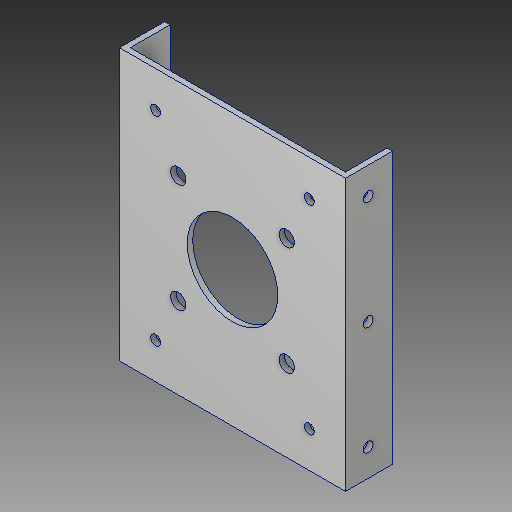
# Autodesk Inventor part: Pneumatic Connector
Saved by Autodesk Inventor 2019 (Build 230136000, 136)
## iProperties
Created: 2019-10-25
Part Number: Pneumatic Connector
Material: Aluminum 6061
Document SubType Name: Modeling
Designer: Mark
Density: 2.7 g/cm^3
Appearance: Aluminum - Flat
Mass: 129.385 g
Surface Area: 498.83 cm^2
Volume: 47.9204 cm^3
Author: Mark
Autodesk Inventor part; units mm, degrees
ref_plane "YZ Plane" through (0, 0, 0) normal (1, 0, 0) x (0, 1, 0)
ref_plane "XZ Plane" through (0, 0, 0) normal (0, 1, 0) x (-1, 0, 0)
ref_plane "XY Plane" through (0, 0, 0) normal (0, 0, 1) x (1, 0, 0)
sketch "Sketch1" plane through (0, 0, 0) normal (0, 1, 0) x (-1, 0, 0)
  line L0 (0, 0) -> (125, 0)
  line L1 (0, 0) -> (125, 0) construction
  line L2 (125, 0) -> (125, -25)
  line L3 (125, -25) -> (122, -25)
  line L4 (122, -25) -> (122, -3)
  line L5 (122, -3) -> (3, -3)
  line L6 (3, -3) -> (3, -26)
  line L7 (3, -26) -> (0, -26)
  line L8 (0, -26) -> (0, 0)
  dimension "d0" = 125
  dimension "d2" = 25
  dimension "d3" = 90
  dimension "d4" = 90
  dimension "d5" = 3
  dimension "d6" = 22
  dimension "d7" = 119
  dimension "d8" = 90
  dimension "d9" = 23
  dimension "d10" = 90
  dimension "d11" = 3
  dimension "d12" = 90
  constraints: 18 end point, 4 perpendicular, 2 horizontal, 1 collinear, 1 vertical
  measures "d0" distance of L0.start L0.end
  measures "d2" distance of L0.end L2.end
  measures "d3" angle of L0 L2
  measures "d4" angle of L3 L2
  measures "d5" distance of L2.end L3.end
  measures "d6" distance of L3.end L4.end
  measures "d7" distance of L4.end L5.end
  measures "d8" angle of L5 L4
  measures "d9" distance of L5.end L6.end
  measures "d10" angle of L6 L5
  measures "d11" distance of L6.end L7.end
  measures "d12" angle of L6 L7
extrude "Extrusion1" add sketch "Sketch1" along normal blind 150
sketch "Sketch2" plane through (-125, 0, 0) normal (0, 0, 1) x (1, 0, 0)
  circle A0 centre (32.5, 105) radius 4.25
  circle A1 centre (92.5, 105) radius 4.25
  circle A2 centre (32.5, 45) radius 4.25
  circle A3 centre (92.5, 45) radius 4.25
  line L0 (125, 0) -> (125, 150) projected
  line L1 (125, 0) -> (0, 0) projected
  circle A4 centre (62.5, 75) radius 25
  dimension "d15" = 8.5
  dimension "d16" = 8.5
  dimension "d17" = 8.5
  dimension "d18" = 8.5
  dimension "d19" = 60
  dimension "d20" = 60
  dimension "d21" = 60
  dimension "d22" = 60
  dimension "d23" = 60
  dimension "d24" = 60
  dimension "d25" = 32.5
  dimension "d26" = 45
  dimension "d27" = 50
  dimension "d28" = 62.5
  dimension "d29" = 75
  constraints: 5 centre point
  measures "d15" diameter of A0
  measures "d16" diameter of A1
  measures "d17" diameter of A2
  measures "d18" diameter of A3
  measures "d19" distance of A0.centre A1.centre
  measures "d20" distance of A3.centre A1.centre
  measures "d21" horizontal distance of A1.centre A2.centre
  measures "d22" distance of A2.centre A3.centre
  measures "d23" distance of A2.centre A0.centre
  measures "d24" horizontal distance of A3.centre A0.centre
  measures "d25" distance from line of L0 A1.centre
  measures "d26" distance from line of L1 A3.centre
  measures "d27" diameter of A4
  measures "d28" distance from line of L0 A4.centre
  measures "d29" distance from line of L1 A4.centre
extrude "Extrusion2" cut sketch "Sketch2" against normal blind 10
sketch "Sketch3" plane through (-125, 0, -25) normal (-1, 0, 0) x (0, 0, 1)
  circle A0 centre (12.5, 15) radius 2.75
  circle A1 centre (12.5, 135) radius 2.75
  line L0 (25, 0) -> (0, 0) projected
  line L1 (0, 150) -> (25, 150) projected
  line L2 (0, 0) -> (0, 150) projected
  line L3 (25, 0) -> (25, 150) projected
  circle A2 centre (12.5, 75) radius 2.75
  dimension "d32" = 5.5
  dimension "d33" = 5.5
  dimension "d34" = 15
  dimension "d35" = 15
  dimension "d36" = 12.5
  dimension "d37" = 12.5
  dimension "d38" = 5.5
  dimension "d39" = 12.5
  dimension "d40" = 75
  constraints: 3 centre point
  measures "d32" diameter of A0
  measures "d33" diameter of A1
  measures "d34" distance from line of L0 A0.centre
  measures "d35" distance from line of L1 A1.centre
  measures "d36" distance from line of L2 A1.centre
  measures "d37" distance from line of L3 A0.centre
  measures "d38" diameter of A2
  measures "d39" distance from line of L3 A2.centre
  measures "d40" distance from line of L0 A2.centre
extrude "Extrusion3" cut sketch "Sketch3" against normal blind 154.4625 contours A0 | A1 | A2
sketch "Sketch5" plane through (-125, 0, 0) normal (0, 0, 1) x (1, 0, 0)
  circle A0 centre (20, 130) radius 2.75
  circle A1 centre (105, 130) radius 2.75
  circle A2 centre (105, 20) radius 2.75
  circle A3 centre (20, 20) radius 2.75
  line L0 (0, 0) -> (0, 150) projected
  line L1 (0, 150) -> (125, 150) projected
  line L2 (125, 0) -> (125, 150) projected
  line L3 (125, 0) -> (0, 0) projected
  dimension "d45" = 5.5
  dimension "d46" = 5.5
  dimension "d47" = 5.5
  dimension "d48" = 5.5
  dimension "d49" = 20
  dimension "d50" = 20
  dimension "d51" = 20
  dimension "d52" = 20
  dimension "d53" = 20
  dimension "d54" = 20
  dimension "d55" = 20
  dimension "d56" = 20
  constraints: 4 centre point
  measures "d45" diameter of A0
  measures "d46" diameter of A1
  measures "d47" diameter of A2
  measures "d48" diameter of A3
  measures "d49" distance from line of L0 A0.centre
  measures "d50" distance from line of L1 A0.centre
  measures "d51" distance from line of L1 A1.centre
  measures "d52" distance from line of L2 A1.centre
  measures "d53" distance from line of L2 A2.centre
  measures "d54" distance from line of L3 A2.centre
  measures "d55" distance from line of L3 A3.centre
  measures "d56" distance from line of L0 A3.centre
extrude "Extrusion5" cut sketch "Sketch5" against normal through all contours A0 | A1 | A2 | A3
equation "\"d50\" = d49"
equation "\"d51\" = d49"
equation "\"d52\" = d49"
equation "\"d53\" = d49"
equation "\"d54\" = d49"
equation "\"d55\" = d49"
equation "\"d56\" = d49"
body "Solid1"
